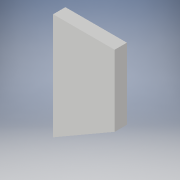
# Autodesk Inventor part: bottom door
Saved by Autodesk Inventor 2017 (Build 210142000, 142)
## iProperties
Created: 2018-03-10
Part Number: bottom door
Material: Generic
Document SubType Name: Modeling
Designer: Braxton
Density: 1 g/cm^3
Appearance: Default
Author: Braxton
Autodesk Inventor part; units mm, degrees
ref_plane "YZ Plane" through (0, 0, 0) normal (1, 0, 0) x (0, 1, 0)
ref_plane "XZ Plane" through (0, 0, 0) normal (0, 1, 0) x (-1, 0, 0)
ref_plane "XY Plane" through (0, 0, 0) normal (0, 0, 1) x (1, 0, 0)
sketch "Sketch1" plane through (0, 0, 0) normal (0, 0, 1) x (1, 0, 0)
  line L0 (1270, 1270) -> (0, 536.7652)
  line L1 (1270, 1270) -> (1270, 2736.4697)
  line L2 (1270, 2736.4697) -> (0, 2736.4697)
  line L3 (0, 2736.4697) -> (0, 536.7652)
  constraints: 8 end point, 1 horizontal, 1 perpendicular
extrude "door" add sketch "Sketch1" along normal mid plane 254
body "Solid1"
